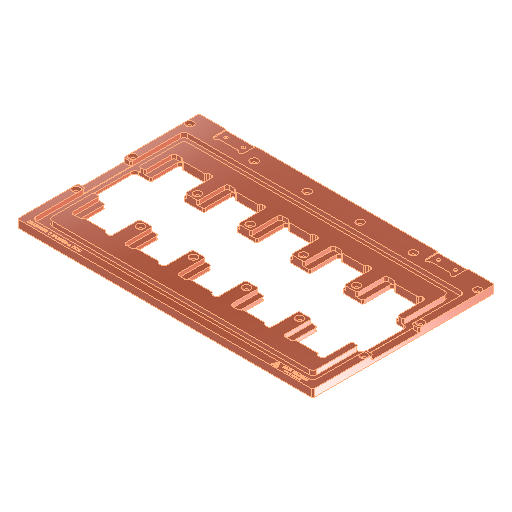
# Autodesk Inventor part: GRJ-04-104
Saved by Autodesk Inventor 2026.1 (Build 301233000, 233)
## iProperties
Company: Gree
Created: 2025-09-10
Part Number: GRJ-04-104
Material: Fenolite OR
Document SubType Name: Modeling
Designer: Willian Pinheiro
Density: 1.38 g/cm^3
Appearance: Suave - Laranja claro
Description: Suporte Dissipador G GRJW890-A
Project: GRJ-04
Mass: 640.909 g
Surface Area: 1542.93 cm^2
Volume: 464.426 cm^3
Checked By: Antonio Lucas
Engr Approved By: Antonio Lucas
Mfg Approved By: Anderson Oliveira
Total: 1
Dimensões: 10 x 240 x 390 mm
Author: Willian Pinheiro
Title: Pasta Dissipador G
Revision Number: 00
Autodesk Inventor part; units mm, degrees
(part 1 of 3)
sketch "comp_ipm-d5-g1-db2" plane through (0, 0, 0) normal (0, 0, 1) x (1, 0, 0)
  line L0 (114.3417, -62.3123) -> (114.3417, -51.4863) construction
  line L1 (114.3417, -51.4863) -> (133.7146, -51.4863) construction
  line L2 (133.611, -89.7496) -> (133.611, -119.2687) construction
  line L3 (133.611, -119.2687) -> (119.4922, -119.2687) construction
  line L4 (119.4922, -119.2687) -> (119.4922, -89.8381) construction
  line L5 (119.4922, -89.8381) -> (119.5805, -89.7496) construction
  line L6 (119.5805, -89.7496) -> (133.611, -89.7496) construction
  line L7 (122.7317, -8.8892) -> (130.2416, -8.8892) construction
  line L8 (133.3346, -81.6323) -> (111.2285, -81.6323) construction
  line L9 (111.2285, -81.6323) -> (111.2285, -65.8863) construction
  line L10 (111.2285, -65.8863) -> (133.3346, -65.8863) construction
  line L11 (133.3346, -65.8863) -> (133.3346, -81.6323) construction
  line L12 (130.2416, -8.8892) -> (130.2416, -41.4312) construction
  line L13 (130.2416, -41.4312) -> (122.7296, -41.4312) construction
  circle A0 centre (120.8945, -10.3261) radius 5 construction
  circle A1 centre (120.8747, -40.1261) radius 5 construction
  arc A2 (122.7096, -57.0141) -> (122.7172, -56.7385) centre (127.7095, -57.0141) ccw construction
  circle A3 centre (127.6714, -73.8746) radius 5 construction
  circle A4 centre (124.6717, -104.6746) radius 5 construction
  line L14 (122.7296, -41.4312) -> (122.7296, -40.059) construction
  arc A5 (122.7296, -40.0576) -> (119.2755, -40.047) centre (121.0027, -40.0154) ccw construction
  line L15 (119.2755, -40.047) -> (119.2755, -41.4312) construction
  line L16 (119.2755, -41.4312) -> (112.2015, -41.4312) construction
  line L17 (112.2015, -41.4312) -> (112.2015, -8.8892) construction
  line L18 (112.2015, -8.8892) -> (119.2755, -8.8892) construction
  line L19 (119.2755, -8.8892) -> (119.2755, -10.254) construction
  arc A6 (119.2755, -10.254) -> (119.2755, -10.1681) centre (121.0022, -10.211) ccw construction
  line L20 (122.7317, -10.1612) -> (122.7317, -8.8892) construction
  circle A7 centre (127.8416, -56.8993) radius 5.127 construction
  line L21 (133.7146, -51.4863) -> (133.7146, -62.3123) construction
  line L22 (133.7146, -62.3123) -> (114.3417, -62.3123) construction
sketch "dissi-g-grjw890-a(v1.6)" plane through (0, 0, 0) normal (0, 0, 1) x (1, 0, 0)
  line L0 (-21.5, -6.5) -> (-21.5, 123.5) construction
  line L1 (31, -6.5) -> (-21.5, -6.5) construction
  line L2 (-21.5, -1.5) -> (31, -1.5) construction
  line L3 (31, -4.5) -> (-21.5, -4.5) construction
  line L4 (31, -6.5) -> (31, 123.5) construction
  line L5 (-21.5, 121.5) -> (31, 121.5) construction
  line L6 (20.379, 118.5) -> (-21.5, 118.5) construction
  line L7 (31, 118.5) -> (23.621, 118.5) construction
  arc A0 (23.621, 118.5) -> (20.379, 118.5) centre (22, 118.5) ccw construction
  arc A1 (20.379, 118.5) -> (23.621, 118.5) centre (22, 118.5) ccw construction
  line L8 (-21.5, 123.5) -> (31, 123.5) construction
  circle A2 centre (9.1772, 15.1514) radius 1.2295 construction
  circle A3 centre (12.177, 45.9515) radius 1.2295 construction
  circle A4 centre (12.3472, 62.9268) radius 1.2295 construction
  circle A5 centre (5.5082, 79.8107) radius 1.2295 construction
  circle A6 centre (5.4, 109.5) radius 1.2295 construction
  arc A7 (0, 71.9528) -> (-1.2857, 75.3) centre (-5, 71.9528) ccw construction
  line L9 (0, 71.9528) -> (0, 0) construction
  line L10 (0, 0) -> (19.4, 0) construction
  line L11 (19.4, 0) -> (19.4, 69.7008) construction
  arc A8 (19.4, 69.7008) -> (17.4571, 71.7) centre (17.4, 69.7008) ccw construction
  arc A9 (12.6, 76.698) -> (17.4571, 71.7) centre (17.6, 76.698) ccw construction
  line L12 (12.6, 76.698) -> (12.6, 113.5) construction
  line L13 (12.6, 113.5) -> (-1.8, 113.5) construction
  line L14 (-1.8, 113.5) -> (-1.8, 76.6389) construction
  arc A10 (-1.8, 76.6389) -> (-1.2857, 75.3) centre (0.2, 76.6389) ccw construction
  circle A11 centre (5.4, 109.5) radius 1.2295 construction
  circle A12 centre (5.5082, 79.8107) radius 1.2295 construction
  line L15 (-14, 123.5) -> (-14, -6.5) construction
  line L16 (28.5, 123.5) -> (28.5, -6.5) construction
  line L17 (-21.5, 58.5) -> (31, 58.5) construction
  line L18 (-1.1528, 57.5138) -> (-1.1528, 68.3398) construction
  line L19 (-1.1528, 68.3398) -> (18.2202, 68.3398) construction
  line L20 (18.1165, 30.0765) -> (18.1165, 0.5573) construction
  line L21 (18.1165, 0.5573) -> (3.9977, 0.5573) construction
  line L22 (3.9977, 0.5573) -> (3.9977, 29.988) construction
  line L23 (3.9977, 29.988) -> (4.0861, 30.0765) construction
  line L24 (4.0861, 30.0765) -> (18.1165, 30.0765) construction
  line L25 (7.2372, 110.9369) -> (14.7471, 110.9369) construction
  line L26 (17.8402, 38.1938) -> (-4.266, 38.1938) construction
  line L27 (-4.266, 38.1938) -> (-4.266, 53.9398) construction
  line L28 (-4.266, 53.9398) -> (17.8402, 53.9398) construction
  line L29 (17.8402, 53.9398) -> (17.8402, 38.1938) construction
  line L30 (14.7471, 110.9369) -> (14.7471, 78.3949) construction
  line L31 (14.7471, 78.3949) -> (7.2352, 78.3949) construction
  circle A13 centre (5.4, 109.5) radius 5 construction
  circle A14 centre (5.3802, 79.6999) radius 5 construction
  arc A15 (7.2151, 62.812) -> (7.2227, 63.0876) centre (12.2151, 62.812) ccw construction
  circle A16 centre (12.177, 45.9515) radius 5 construction
  circle A17 centre (9.1772, 15.1514) radius 5 construction
  line L32 (7.2352, 78.3949) -> (7.2352, 79.7671) construction
  arc A18 (7.2352, 79.7685) -> (3.781, 79.779) centre (5.5082, 79.8107) ccw construction
  line L33 (3.781, 79.779) -> (3.781, 78.3949) construction
  line L34 (3.781, 78.3949) -> (-3.293, 78.3949) construction
  line L35 (-3.293, 78.3949) -> (-3.293, 110.9369) construction
  line L36 (-3.293, 110.9369) -> (3.781, 110.9369) construction
  line L37 (3.781, 110.9369) -> (3.781, 109.5721) construction
  arc A19 (3.781, 109.5721) -> (3.781, 109.658) centre (5.5077, 109.615) ccw construction
  line L38 (7.2372, 109.6648) -> (7.2372, 110.9369) construction
  circle A20 centre (12.3472, 62.9268) radius 5.127 construction
  line L39 (18.2202, 68.3398) -> (18.2202, 57.5138) construction
  line L40 (18.2202, 57.5138) -> (-1.1528, 57.5138) construction
  dimension "d211" = 7.5
  dimension "d212" = 2.5
  measures "d211" distance between parallel lines of L0 L15
  measures "d212" distance between parallel lines of L4 L16
sketch "Logo-Delta" plane through (0, 0, 0) normal (0, 0, 1) x (1, 0, 0)
  line L0 (-108.5421, -93.8239) -> (-105.2306, -99.7477)
  line L1 (-105.8771, -100.8237) -> (-112.693, -100.8237)
  line L2 (-113.3004, -99.7477) -> (-112.693, -100.8237)
  line L3 (-109.8866, -93.8239) -> (-113.3004, -99.7477)
  line L4 (-109.8866, -93.8239) -> (-108.5421, -93.8239)
  line L5 (-108.6943, -94.0618) -> (-109.6978, -94.0618)
  line L6 (-107.1297, -98.6558) -> (-109.869, -98.6558)
  line L7 (-110.3581, -99.4928) -> (-105.6768, -99.4597)
  line L8 (-108.6943, -94.0618) -> (-105.6768, -99.4597)
  line L9 (-107.5019, -98.4356) -> (-108.4992, -98.4356)
  line L10 (-109.8866, -96.0618) -> (-112.5468, -100.5747)
  line L11 (-112.9983, -99.775) -> (-109.8866, -94.3555)
  line L12 (-109.869, -98.6558) -> (-110.3581, -99.4928)
  line L13 (-109.8866, -94.3555) -> (-107.5019, -98.4356)
  line L14 (-109.6978, -94.0618) -> (-109.6206, -94.2)
  line L15 (-109.8866, -96.0618) -> (-108.4992, -98.4356)
  line L16 (-109.6978, -94.0618) -> (-107.1297, -98.6558)
  line L17 (-112.9983, -99.775) -> (-112.5468, -100.5747)
  line L18 (-105.2306, -99.7477) -> (-105.8771, -100.8237)
  line L19 (-109.3597, -97.315) -> (-110.8037, -99.7825)
  line L20 (-110.8037, -99.7825) -> (-105.5116, -99.7553)
  line L21 (-105.5116, -99.7553) -> (-105.978, -100.5522)
  line L22 (-105.978, -100.5522) -> (-112.2705, -100.5522)
  line L23 (-112.2705, -100.5522) -> (-109.8735, -96.4562)
  line L24 (-109.2558, -97.6251) -> (-109.7424, -98.4356)
  line L25 (-109.7424, -98.4356) -> (-108.7692, -98.4356)
  line L26 (-108.7692, -98.4356) -> (-109.2558, -97.6251)
  line L27 (-109.8735, -96.4562) -> (-109.3597, -97.315)
  line L28 (-109.2558, -97.6251) -> (-108.7692, -98.4356)
  point P0 (-109.285, -100.8237)
  dimension "d228" = 33
  dimension "d229" = 50
  dimension "d230" = 5
  dimension "d231" = 9
  dimension "d232" = 2.5
  dimension "d233" = 6
  dimension "d234" = 150
  dimension "d235" = 12
  dimension "d236" = 15
  dimension "d237" = 13.4
  dimension "d238" = 5.5006
  dimension "d239" = 12.9994
  dimension "d240" = 12.9994
  dimension "d227" = 7
sketch "Esboço1" plane through (0, 0, 0) normal (0, 0, 1) x (1, 0, 0)
  line L0 (-195, 130) -> (195, 130)
  line L1 (195, 130) -> (195, -110)
  line L2 (195, -110) -> (-195, -110)
  line L3 (-195, -110) -> (-195, 130)
  line L4 (0, 179.4497) -> (0, -159.4497) construction
  line L5 (-274.4497, 0) -> (274.4497, 0) construction
  arc A0 (-190, 130) -> (-195, 125) centre (-190, 125) ccw
  arc A1 (195, 125) -> (190, 130) centre (190, 125) ccw
  arc A2 (190, -110) -> (195, -105) centre (190, -105) ccw
  arc A3 (-195, -105) -> (-190, -110) centre (-190, -105) ccw
  line L6 (-165, 0) -> (-65, 0) construction
  line L7 (-113.55, 65.2) -> (-166.45, 65.2)
  line L8 (-166.45, 65.2) -> (-166.45, -65.2)
  line L9 (-166.45, -65.2) -> (-113.55, -65.2)
  line L10 (-113.55, -65.2) -> (-113.55, 65.2)
  line L11 (-116.05, 65.2) -> (-158.95, 65.2)
  line L12 (-158.95, 65.2) -> (-158.95, -65.2)
  line L13 (-158.95, -65.2) -> (-116.05, -65.2)
  line L14 (-116.05, -65.2) -> (-116.05, 65.2)
  line L15 (-158.95, 0) -> (-116.05, 0) construction
  line L16 (-195, 30) -> (195, 30)
  line L17 (195, 30) -> (195, -30)
  line L18 (195, -30) -> (-195, -30)
  line L19 (-195, -30) -> (-195, 30)
  line L20 (-175, 90) -> (175, 90) construction
  line L21 (175, 90) -> (175, -90) construction
  line L22 (175, -90) -> (-175, -90) construction
  line L23 (-175, -90) -> (-175, 90) construction
  line L24 (-185, 100) -> (185, 100) construction
  line L25 (185, 100) -> (185, -100) construction
  line L26 (185, -100) -> (-185, -100) construction
  line L27 (-185, -100) -> (-185, 100) construction
  line L28 (185.4, 100.4) -> (-185.4, 100.4)
  line L29 (-185.4, 100.4) -> (-185.4, -100.4)
  line L30 (-185.4, -100.4) -> (185.4, -100.4)
  line L31 (185.4, -100.4) -> (185.4, 100.4)
  line L32 (174.6, 89.6) -> (-174.6, 89.6)
  line L33 (-174.6, 89.6) -> (-174.6, -89.6)
  line L34 (-174.6, -89.6) -> (174.6, -89.6)
  line L35 (174.6, -89.6) -> (174.6, 89.6)
  line L36 (-159.5, 130) -> (-120.5, 130)
  line L37 (-120.5, 130) -> (-120.5, 114)
  line L38 (-120.5, 114) -> (-159.5, 114)
  line L39 (-159.5, 114) -> (-159.5, 130)
  circle A4 centre (-156.5, 114) radius 3
  line L40 (-140, 114) -> (-140, 130) construction
  line L41 (-159.5, 122) -> (-120.5, 122) construction
  circle A5 centre (-123.5, 114) radius 3
  line L42 (159.5, 130) -> (120.5, 130)
  line L43 (120.5, 130) -> (120.5, 114)
  line L44 (120.5, 114) -> (159.5, 114)
  line L45 (159.5, 114) -> (159.5, 130)
  circle A6 centre (156.5, 114) radius 3
  line L46 (140, 114) -> (140, 130) construction
  line L47 (159.5, 122) -> (120.5, 122) construction
  circle A7 centre (123.5, 114) radius 3
  line L48 (-195, 10) -> (195, 10) construction
  line L49 (-180, 30) -> (-180, -30)
  line L50 (180, 30) -> (180, -30)
  line L51 (-140, 65) -> (-140, -65) construction
  line L52 (-105, 89.6) -> (-105, -100.4) construction
  line L53 (-70, 65) -> (-70, -65) construction
  line L54 (140, 65) -> (140, -65) construction
  line L55 (70, 65) -> (70, -65) construction
  circle A8 centre (-163.45, 65.2) radius 3
  circle A9 centre (-119.05, 65.2) radius 3
  circle A10 centre (-155.95, 65.2) radius 3
  circle A11 centre (-116.55, 65.2) radius 3
  circle A12 centre (-163.45, -65.2) radius 3
  circle A13 centre (-119.05, -65.2) radius 3
  circle A14 centre (-155.95, -65.2) radius 3
  circle A15 centre (-116.55, -65.2) radius 3
  line L56 (-163.45, 68.2) -> (-155.95, 68.2)
  line L57 (-116.55, 68.2) -> (-119.05, 68.2)
  line L58 (-163.45, -68.2) -> (-155.95, -68.2)
  line L59 (-119.05, -68.2) -> (-116.55, -68.2)
  line L60 (-166.25, -65) -> (-166.25, 65) construction
  line L61 (-113.75, -65) -> (-166.25, -65) construction
  line L62 (-166.25, -60) -> (-113.75, -60) construction
  line L63 (-113.75, -63) -> (-166.25, -63) construction
  line L64 (-113.75, -65) -> (-113.75, 65) construction
  line L65 (-166.25, 63) -> (-113.75, 63) construction
  line L66 (-124.371, 60) -> (-166.25, 60) construction
  line L67 (-113.75, 60) -> (-121.129, 60) construction
  arc A16 (-121.129, 60) -> (-124.371, 60) centre (-122.75, 60) ccw construction
  arc A17 (-124.371, 60) -> (-121.129, 60) centre (-122.75, 60) ccw construction
  line L68 (-166.25, 65) -> (-113.75, 65) construction
  circle A18 centre (-135.5728, -43.3486) radius 1.2295 construction
  circle A19 centre (-132.573, -12.5485) radius 1.2295 construction
  circle A20 centre (-132.4028, 4.4268) radius 1.2295 construction
  circle A21 centre (-139.2418, 21.3107) radius 1.2295 construction
  circle A22 centre (-139.35, 51) radius 1.2295 construction
  arc A23 (-144.75, 13.4528) -> (-146.0357, 16.8) centre (-149.75, 13.4528) ccw construction
  line L69 (-144.75, 13.4528) -> (-144.75, -58.5) construction
  line L70 (-144.75, -58.5) -> (-125.35, -58.5) construction
  line L71 (-125.35, -58.5) -> (-125.35, 11.2008) construction
  arc A24 (-125.35, 11.2008) -> (-127.2929, 13.2) centre (-127.35, 11.2008) ccw construction
  arc A25 (-132.15, 18.198) -> (-127.2929, 13.2) centre (-127.15, 18.198) ccw construction
  line L72 (-132.15, 18.198) -> (-132.15, 55) construction
  line L73 (-132.15, 55) -> (-146.55, 55) construction
  line L74 (-146.55, 55) -> (-146.55, 18.1389) construction
  arc A26 (-146.55, 18.1389) -> (-146.0357, 16.8) centre (-144.55, 18.1389) ccw construction
  circle A27 centre (-139.35, 51) radius 1.2295 construction
  circle A28 centre (-139.2418, 21.3107) radius 1.2295 construction
  line L75 (-158.75, 65) -> (-158.75, -65) construction
  line L76 (-116.25, 65) -> (-116.25, -65) construction
  line L77 (-166.25, 0) -> (-113.75, 0) construction
  line L78 (-145.9028, -0.9862) -> (-145.9028, 9.8398) construction
  line L79 (-145.9028, 9.8398) -> (-126.5298, 9.8398) construction
  line L80 (-126.6335, -28.4235) -> (-126.6335, -57.9427) construction
  line L81 (-126.6335, -57.9427) -> (-140.7523, -57.9427) construction
  line L82 (-140.7523, -57.9427) -> (-140.7523, -28.512) construction
  line L83 (-140.7523, -28.512) -> (-140.6639, -28.4235) construction
  line L84 (-140.6639, -28.4235) -> (-126.6335, -28.4235) construction
  line L85 (-137.5128, 52.4369) -> (-130.0029, 52.4369) construction
  line L86 (-126.9098, -20.3062) -> (-149.016, -20.3062) construction
  line L87 (-149.016, -20.3062) -> (-149.016, -4.5602) construction
  line L88 (-149.016, -4.5602) -> (-126.9098, -4.5602) construction
  line L89 (-126.9098, -4.5602) -> (-126.9098, -20.3062) construction
  line L90 (-130.0029, 52.4369) -> (-130.0029, 19.8949) construction
  line L91 (-130.0029, 19.8949) -> (-137.5148, 19.8949) construction
  circle A29 centre (-139.35, 51) radius 5 construction
  circle A30 centre (-139.3698, 21.1999) radius 5 construction
  arc A31 (-137.5349, 4.312) -> (-137.5273, 4.5876) centre (-132.5349, 4.312) ccw construction
  circle A32 centre (-132.573, -12.5485) radius 5 construction
  circle A33 centre (-135.5728, -43.3486) radius 5 construction
  line L92 (-137.5148, 19.8949) -> (-137.5148, 21.2671) construction
  arc A34 (-137.5148, 21.2685) -> (-140.969, 21.279) centre (-139.2418, 21.3107) ccw construction
  line L93 (-140.969, 21.279) -> (-140.969, 19.8949) construction
  line L94 (-140.969, 19.8949) -> (-148.043, 19.8949) construction
  line L95 (-148.043, 19.8949) -> (-148.043, 52.4369) construction
  line L96 (-148.043, 52.4369) -> (-140.969, 52.4369) construction
  line L97 (-140.969, 52.4369) -> (-140.969, 51.0721) construction
  arc A35 (-140.969, 51.0721) -> (-140.969, 51.158) centre (-139.2423, 51.115) ccw construction
  line L98 (-137.5128, 51.1648) -> (-137.5128, 52.4369) construction
  circle A36 centre (-132.4028, 4.4268) radius 5.127 construction
  line L99 (-126.5298, 9.8398) -> (-126.5298, -0.9862) construction
  line L100 (-126.5298, -0.9862) -> (-145.9028, -0.9862) construction
  point P0 (0, 0)
  point P1 (-151.5, 122)
  point P2 (-128.5, 122)
  point P3 (151.5, 122)
  point P4 (128.5, 122)
  point P5 (-190, 37.5)
  point P6 (-190, -37.5)
  point P7 (190, 37.5)
  point P8 (190, -37.5)
  point P9 (-190, 112.5)
  point P10 (190, 112.5)
  point P11 (-35, 37.5)
  point P12 (-35, -37.5)
  point P13 (-35, 112.5)
  point P14 (35, 37.5)
  point P15 (35, -37.5)
  point P16 (35, 112.5)
  point P17 (120.5, 114)
  point P18 (126.5, 114)
  point P19 (153.5, 114)
  point P20 (159.5, 130)
  point P21 (120.5, 130)
  point P22 (-120.5, 114)
  point P23 (-120.5, 130)
  point P24 (-153.5, 114)
  point P25 (-126.5, 114)
  point P26 (-185.4, -30)
  point P27 (185.4, -30)
  point P28 (185.4, 30)
  point P29 (-185.4, 30)
  point P30 (-174.6, 30)
  point P31 (-174.6, -30)
  point P32 (174.6, -30)
  point P33 (174.6, 30)
  point P34 (-160.45, -65.2)
  point P35 (-119.55, -65.2)
  point P36 (-119.55, 65.2)
  point P37 (-160.45, 65.2)
  point P38 (-152.95, 65.2)
  point P39 (-152.95, -65.2)
  point P40 (-122.05, -65.2)
  point P41 (-122.05, 65.2)
  point P42 (-105, 37.5)
  point P43 (-105, -37.5)
  point P44 (-105, 112.5)
  point P45 (105, 37.5)
  point P46 (105, 112.5)
  point P47 (105, -37.5)
  dimension "d210" = 6
  dimension "d0" = 390
  dimension "d1" = 240
  dimension "d2" = 5
  dimension "d145" = 110
  dimension "d151" = 60
  dimension "d153" = 20
  dimension "d154" = 20
  dimension "d155" = 40
  dimension "d156" = 10
  dimension "d157" = 0.4
  dimension "d158" = 0.4
  dimension "d159" = 39
  dimension "d160" = 16
  dimension "d161" = 8
  dimension "d162" = 23
  dimension "d163" = 280
  dimension "d164" = 75
  dimension "d165" = 5
  dimension "d166" = 75
  dimension "d167" = 70
  dimension "d218" = 70
  dimension "d219" = 70
  dimension "d220" = 0.2
  dimension "d221" = 0.2
  dimension "d222" = 0.2
  dimension "d223" = 0.2
  constraints: 116 end point, 36 symmetric about line, 24 point on line, 18 parallel, 11 perpendicular, 10 horizontal, 10 midpoint, 8 point on circle, 8 tangent, 7 vertical alignment, 6 centre point, 5 vertical, 3 collinear, 3 equal radius, 3 horizontal alignment, 50 other
  measures "d0" distance of L0.start L0.end
  measures "d1" distance of L0.start L2.end
  measures "d2" radius of A0
  measures "d145" distance between parallel lines of L2 L5
  measures "d151" distance between parallel lines of L18 L16
  measures "d153" distance between parallel lines of L23 L3
  measures "d154" distance between parallel lines of L2 L22
  measures "d155" distance between parallel lines of L20 L0
  measures "d156" distance between parallel lines of L23 L27
  measures "d157" distance between parallel lines of L31 L25
  measures "d158" distance between parallel lines of L21 L35
  measures "d159" distance between parallel lines of L37 L39
  measures "d160" distance between parallel lines of L0 L38
  measures "d161" distance between parallel lines of L41 L36
  measures "d162" distance of point (-128.5, 122) point (-151.5, 122)
  measures "d163" distance between parallel lines of L40 L46
  measures "d164" distance of point (-190, 37.5) point (-190, -37.5)
  measures "d165" distance from line of L3 point (-190, -37.5)
  measures "d166" distance of point (-190, 112.5) point (-190, 37.5)
  measures "d167" distance of point (35, 112.5) point (-35, 112.5)
  measures "d218" distance between parallel lines of L4 L53
  measures "d219" distance between parallel lines of L51 L53
extrude "Extrusão1" add sketch "Esboço1" against normal blind 10
extrude "Extrusion22" cut sketch "Esboço1" against normal blind 1.3 contours L0 L37 A5 L38 A4 L39 | A4 L38 | L38 A4 | L0 L45 A6 L44 A7 L43 | A5 L38 | L38 A5 | A7 L44 | L44 A7 | A6 L44 | L44 A6
extrude "Extrusion23" cut sketch "Esboço1" against normal blind 6.1 contours L29 L28 L31 L16 L35 L32 L33 | L16 L49 L18 L29 | L18 L33 L34 L35 L31 L30 L29 | L16 L33 L18 L49 | L31 L18 L50 L16 | L50 L18 L35 L16
extrude "Extrusion24" cut sketch "Esboço1" against normal blind 5.4 contours L16 L29 L18 L3 | L16 L12 L18 L8 | L8 A8 L7 L12 L16 | L16 L1 L18 L31 | L18 L12 L9 A12 L8 | A8 L7 | L7 A8 | L16 L14 L18 L12 | L12 A10 L7 A9 A11 L14 L16 | A12 L9 | L9 A12 | L18 L14 A15 A13 L9 A14 L12 | A8 L56 A10 L7 | A10 L7 | L7 A10 | L16 L10 L18 L14 | L14 A11 L10 L16 | L9 A14 L58 A12 | A14 L9 | L9 A14 | L18 L10 A15 L14 | A11 A9 L14 | L14 L7 A11 | A15 L9 L14 | L14 A13 A15 | A9 A11 L7 | L7 A11 A9 | A9 A11 L7 | A9 A11 L7 | L7 A11 A9 | A13 A15 L9 | L9 A15 A13 | A13 A15 L9 | L9 A15 A13 | L9 A15 A13 | L57 A11 A9 | A13 A15 L59
extrude "Extrusion25" cut sketch "Esboço1" against normal through all contours L16 L14 L18 L12 | L12 A10 L7 A9 A11 L14 L16 | L18 L14 A15 A13 L9 A14 L12 | A10 L7 | L7 A10 | A14 L9 | L9 A14 | A11 A9 L14 | L14 A13 A15 | A9 A11 L7 | L7 A11 A9 | A9 A11 L7 | L7 A11 A9 | A13 A15 L9 | L9 A15 A13 | A13 A15 L9 | L9 A15 A13 picked at (-120.3323, 65.6487) picked at (-120.3328, 64.7533) picked at (-117.2426, 64.9738) picked at (-117.2426, 65.4262) picked at (-120.3328, -64.7533) picked at (-120.3323, -65.6487) picked at (-118.3574, -65.4262) picked at (-117.2426, -64.9738)
pattern_linear "Rectangular Pattern4" count 5 spacing 70 along (1, 0, 0) of "Extrusion24", "Extrusion25"
extrude "Extrusion26" cut sketch "Esboço1" against normal through all contours L16 L33 L18 L49 | L16 L8 L18 L33 | L16 L12 L18 L8 | L16 L14 L18 L12 | L50 L18 L35 L16 | L16 L10 L18 L14 | L35 L18 L10 L16
hole "Hole3" at (-151.5, 122, 0) at (-128.5, 122, 0) at (128.5, 122, 0) at (151.5, 122, 0) direction (0, 0, -1) diameter 2.459 end through all thread size "M3x0.5" class "6H" standard "ISO Metric profile"
hole "Hole4" at (-190, 37.5, 0) at (-190, -37.5, 0) at (190, 37.5, 0) at (190, -37.5, 0) at (-190, 112.5, 0) at (190, 112.5, 0) at (-35, 37.5, 0) at (-35, -37.5, 0) at (-35, 112.5, 0) at (35, 37.5, 0) at (35, 112.5, 0) at (35, -37.5, 0) at (-105, 112.5, 0) at (-105, 37.5, 0) at (-105, -37.5, 0) at (105, -37.5, 0) at (105, 37.5, 0) at (105, 112.5, 0) direction (0, 0, -1) diameter 4.5 end through all countersink diameter 10 countersink angle 90 clearance for "Countersunk Flat Head Hex Socket Screw ISO 10642" size "M4" standard "ISO"
fillet "Fillet10" radius 2 84 edges at (-113.55, 30, -2.7) (-96.45, 30, -2.7) (-113.55, -30, -2.7) (-96.45, -30, -2.7) (-43.55, 30, -2.7) (-26.45, 30, -2.7) (-26.45, -30, -2.7) (-43.55, -30, -2.7) (26.45, -30, -2.7) (174.6, -30, -3.05) (174.6, 30, -3.05) (26.45, 30, -2.7) (-166.45, -30, -2.7) (-174.6, -30, -3.05) (-153.5, 114, -0.65) (-126.5, 114, -0.65) (126.5, 114, -0.65) (153.5, 114, -0.65) (-174.6, 30, -3.05) (-166.45, 30, -2.7) (-195, 30, -2.7) (-185.4, 30, -2.7) (-195, -30, -2.7) (-185.4, -30, -2.7) (185.4, 30, -2.7) (195, 30, -2.7) (185.4, -30, -2.7) (195, -30, -2.7) (195, 130, -5) (195, -110, -5) (-195, -110, -5) (-195, 130, -5) (-152.95, 65.2, -5) (-122.05, 65.2, -5) (-116.05, 30, -7.7) (-158.95, 30, -7.7) (-88.95, 30, -7.7) (-82.95, 65.2, -5) (-52.05, 65.2, -5) (-46.05, 30, -7.7) (-18.95, 30, -7.7) (-12.95, 65.2, -5) (17.95, 65.2, -5) (23.95, 30, -7.7) (51.05, 30, -7.7) (57.05, 65.2, -5) (87.95, 65.2, -5) (93.95, 30, -7.7) (96.45, 30, -2.7) (43.55, 30, -2.7) (113.55, 30, -2.7) (121.05, 30, -7.7) (127.05, 65.2, -5) (157.95, 65.2, -5) (163.95, 30, -7.7) (166.45, 30, -2.7) (166.45, -30, -2.7) (163.95, -30, -7.7) (113.55, -30, -2.7) (121.05, -30, -7.7) (93.95, -30, -7.7) (96.45, -30, -2.7) (127.05, -65.2, -5) (157.95, -65.2, -5) (87.95, -65.2, -5) (57.05, -65.2, -5) (51.05, -30, -7.7) (43.55, -30, -2.7) (23.95, -30, -7.7) (17.95, -65.2, -5) (-12.95, -65.2, -5) (-18.95, -30, -7.7) (-46.05, -30, -7.7) (-88.95, -30, -7.7) (-116.05, -30, -7.7) (-158.95, -30, -7.7) (-152.95, -65.2, -5) (-122.05, -65.2, -5) (-82.95, -65.2, -5) (-52.05, -65.2, -5) (-159.5, 130, -0.65) (-120.5, 130, -0.65) (120.5, 130, -0.65) (159.5, 130, -0.65)
fillet "Fillet10" radius 5 12 edges at (174.6, -89.6, -3.05) (185.4, -100.4, -3.05) (-185.4, -100.4, -3.05) (-174.6, -89.6, -3.05) (-185.4, 100.4, -3.05) (-174.6, 89.6, -3.05) (185.4, 100.4, -3.05) (174.6, 89.6, -3.05) (-180, 30, -8.05) (-180, -30, -8.05) (180, -30, -8.05) (180, 30, -8.05)
chamfer "Chamfer3" [suppressed]
chamfer "Chamfer4" distance 1 angle 45 4 edges at (-151.5, 123.2295, -1.3) (-128.5, 123.2295, -1.3) (128.5, 123.2295, -1.3) (151.5, 123.2295, -1.3)
ref_plane "Work Plane1" through (-140, 65.2, 0) normal (1, 0, 0) x (0, 0, -1)
ref_plane "Work Plane2" through (-70, 65.2, 0) normal (1, 0, 0) x (0, 0, -1)
ref_plane "Work Plane3" through (0, 65.2, 0) normal (1, 0, 0) x (0, 0, -1)
ref_plane "Plano de trabalho4" through (70, 65.2, 0) normal (1, 0, 0) x (0, 0, -1)
ref_plane "Plano de trabalho5" through (140, 65.2, 0) normal (1, 0, 0) x (0, 0, -1)
sketch "Esboço27" plane through (0, 0, 0) normal (0, 0, 1) x (1, 0, 0)
  line L0 (-185.4, -107) -> (-185.4, -103) construction
  line L1 (-185.4, -103) -> (-2.1339, -103) construction
  line L2 (-2.1339, -103) -> (-2.1339, -107) construction
  line L3 (-2.1339, -107) -> (-185.4, -107) construction
  line L4 (-193, -110) -> (193, -110) projected
  line L5 (-195, -37.5) -> (-195, -108) projected
  line L6 (145.4, -108.5) -> (145.4, -101.5) construction
  line L7 (148.9, -108.5) -> (148.9, -104.5) construction
  line L8 (165.4, -101.5) -> (165.4, -108.5) construction
  line L9 (181.9, -104.5) -> (181.9, -108.5) construction
  line L10 (148.9, -104.5) -> (181.9, -104.5) construction
  line L11 (181.9, -108.5) -> (148.9, -108.5) construction
  line L12 (185.4, -108.5) -> (145.4, -108.5) construction
  line L13 (185.4, -101.5) -> (185.4, -108.5) construction
  line L14 (145.4, -101.5) -> (185.4, -101.5) construction
  line L15 (185.4, -39.4596) -> (185.4, -95.4) construction
  line L16 (-185.4, -95.4) -> (-185.4, -39.4596) projected
  line L17 (143.0723, -101.5) -> (146.3837, -107.4238)
  line L18 (145.7373, -108.4998) -> (138.9214, -108.4998)
  line L19 (138.3139, -107.4238) -> (138.9214, -108.4998)
  line L20 (141.7277, -101.5) -> (138.3139, -107.4238)
  line L21 (141.7277, -101.5) -> (143.0723, -101.5)
  line L22 (142.9201, -101.7378) -> (141.9165, -101.7378)
  line L23 (144.4846, -106.3319) -> (141.7453, -106.3319)
  line L24 (141.2562, -107.1689) -> (145.9375, -107.1357)
  line L25 (142.9201, -101.7378) -> (145.9375, -107.1357)
  line L26 (144.1124, -106.1117) -> (143.1151, -106.1117)
  line L27 (141.7277, -103.7379) -> (139.0676, -108.2507)
  line L28 (138.6161, -107.451) -> (141.7277, -102.0316)
  line L29 (141.7453, -106.3319) -> (141.2562, -107.1689)
  line L30 (141.7277, -102.0316) -> (144.1124, -106.1117)
  line L31 (141.9165, -101.7378) -> (141.9938, -101.8761)
  line L32 (141.7277, -103.7379) -> (143.1151, -106.1117)
  line L33 (141.9165, -101.7378) -> (144.4846, -106.3319)
  line L34 (138.6161, -107.451) -> (139.0676, -108.2507)
  line L35 (146.3837, -107.4238) -> (145.7373, -108.4998)
  line L36 (142.2546, -104.991) -> (140.8106, -107.4586)
  line L37 (140.8106, -107.4586) -> (146.1027, -107.4314)
  line L38 (146.1027, -107.4314) -> (145.6364, -108.2283)
  line L39 (145.6364, -108.2283) -> (139.3439, -108.2283)
  line L40 (139.3439, -108.2283) -> (141.7409, -104.1323)
  line L41 (142.3585, -105.3012) -> (141.8719, -106.1117)
  line L42 (141.8719, -106.1117) -> (142.8452, -106.1117)
  line L43 (142.8452, -106.1117) -> (142.3585, -105.3012)
  line L44 (141.7409, -104.1323) -> (142.2546, -104.991)
  line L45 (142.3585, -105.3012) -> (142.8452, -106.1117)
  spline S0 degree 2 poles (-185.0494, -103.5227) (-185.0494, -103.3474) (-184.874, -103.3474) knots 0 0 0 1 1 1
  line L46 (-184.874, -103.3474) -> (-183.8253, -103.3474)
  spline S1 degree 2 poles (-183.8253, -103.3474) (-183.4584, -103.3474) (-182.9519, -103.8539) (-182.9519, -104.2208) knots 0 0 0 1 2 2 2
  line L47 (-182.9519, -104.2208) -> (-182.9519, -105.9708)
  spline S2 degree 2 poles (-182.9519, -105.9708) (-182.9519, -106.3344) (-183.4617, -106.8474) (-183.8253, -106.8474) knots 0 0 0 1 2 2 2
  line L48 (-183.8253, -106.8474) -> (-184.874, -106.8474)
  spline S3 degree 2 poles (-184.874, -106.8474) (-185.0494, -106.8474) (-185.0494, -106.6721) knots 0 0 0 1 1 1
  line L49 (-185.0494, -106.6721) -> (-185.0494, -103.5227)
  line L50 (-184.6987, -103.6981) -> (-184.6987, -106.4968)
  line L51 (-184.6987, -106.4968) -> (-183.8253, -106.4968)
  spline S4 degree 2 poles (-183.8253, -106.4968) (-183.6078, -106.4968) (-183.3026, -106.1883) (-183.3026, -105.9708) knots 0 0 0 1 2 2 2
  line L52 (-183.3026, -105.9708) -> (-183.3026, -104.224)
  spline S5 degree 2 poles (-183.3026, -104.224) (-183.3026, -104.0065) (-183.6078, -103.6981) (-183.8253, -103.6981) knots 0 0 0 1 2 2 2
  line L53 (-183.8253, -103.6981) -> (-184.6987, -103.6981)
  spline S6 degree 2 poles (-182.0753, -106.8474) (-182.2506, -106.8474) (-182.2506, -106.6721) knots 0 0 0 1 1 1
  line L54 (-182.2506, -106.6721) -> (-182.2506, -103.5227)
  spline S7 degree 2 poles (-182.2506, -103.5227) (-182.2506, -103.3474) (-182.0753, -103.3474) knots 0 0 0 1 1 1
  spline S8 degree 2 poles (-182.0753, -103.3474) (-181.9, -103.3474) (-181.9, -103.5227) knots 0 0 0 1 1 1
  line L55 (-181.9, -103.5227) -> (-181.9, -106.6721)
  spline S9 degree 2 poles (-181.9, -106.6721) (-181.9, -106.8474) (-182.0753, -106.8474) knots 0 0 0 1 1 1
  spline S10 degree 2 poles (-179.1045, -105.974) (-179.1045, -106.3344) (-179.6175, -106.8474) (-179.9779, -106.8474) knots 0 0 0 1 2 2 2
  spline S11 degree 2 poles (-179.9779, -106.8474) (-180.624, -106.8474) (-181.124, -106.4643) knots 0 0 0 1 1 1
  spline S12 degree 2 poles (-181.124, -106.4643) (-181.2019, -106.4058) (-181.2019, -106.3214) knots 0 0 0 1 1 1
  spline S13 degree 2 poles (-181.2019, -106.3214) (-181.2019, -106.25) (-181.0981, -106.1461) (-181.0266, -106.1461) knots 0 0 0 1 2 2 2
  spline S14 degree 2 poles (-181.0266, -106.1461) (-180.9844, -106.1461) (-180.926, -106.1786) knots 0 0 0 1 1 1
  spline S15 degree 2 poles (-180.926, -106.1786) (-180.7734, -106.2727) (-180.4455, -106.4221) knots 0 0 0 1 1 1
  spline S16 degree 2 poles (-180.4455, -106.4221) (-180.2312, -106.4968) (-179.9779, -106.4968) knots 0 0 0 1 1 1
  spline S17 degree 2 poles (-179.9779, -106.4968) (-179.7636, -106.4968) (-179.4552, -106.1883) (-179.4552, -105.9708) knots 0 0 0 1 2 2 2
  spline S18 degree 2 poles (-179.4552, -105.9708) (-179.4552, -105.6526) (-179.7474, -105.5032) knots 0 0 0 1 1 1
  line L56 (-179.7474, -105.5032) -> (-180.7279, -105)
  spline S19 degree 2 poles (-180.7279, -105) (-181.2019, -104.7565) (-181.2019, -104.2208) knots 0 0 0 1 1 1
  spline S20 degree 2 poles (-181.2019, -104.2208) (-181.2019, -103.8604) (-180.689, -103.3474) (-180.3286, -103.3474) knots 0 0 0 1 2 2 2
  spline S21 degree 2 poles (-180.3286, -103.3474) (-179.7084, -103.3474) (-179.3838, -103.539) knots 0 0 0 1 1 1
  spline S22 degree 2 poles (-179.3838, -103.539) (-179.2799, -103.6006) (-179.2799, -103.6981) knots 0 0 0 1 1 1
  spline S23 degree 2 poles (-179.2799, -103.6981) (-179.2799, -103.7695) (-179.3838, -103.8734) (-179.4552, -103.8734) knots 0 0 0 1 2 2 2
  spline S24 degree 2 poles (-179.4552, -103.8734) (-179.4812, -103.8734) (-179.5299, -103.8539) knots 0 0 0 1 1 1
  spline S25 degree 2 poles (-179.5299, -103.8539) (-179.9325, -103.6981) (-180.3286, -103.6981) knots 0 0 0 1 1 1
  spline S26 degree 2 poles (-180.3286, -103.6981) (-180.5461, -103.6981) (-180.8513, -104.0065) (-180.8513, -104.224) knots 0 0 0 1 2 2 2
  spline S27 degree 2 poles (-180.8513, -104.224) (-180.8513, -104.5422) (-180.5656, -104.6883) knots 0 0 0 1 1 1
  line L57 (-180.5656, -104.6883) -> (-179.5851, -105.1916)
  spline S28 degree 2 poles (-179.5851, -105.1916) (-179.1045, -105.4383) (-179.1045, -105.974) knots 0 0 0 1 1 1
  spline S29 degree 2 poles (-176.3058, -105.974) (-176.3058, -106.3344) (-176.8188, -106.8474) (-177.1792, -106.8474) knots 0 0 0 1 2 2 2
  spline S30 degree 2 poles (-177.1792, -106.8474) (-177.8253, -106.8474) (-178.3253, -106.4643) knots 0 0 0 1 1 1
  spline S31 degree 2 poles (-178.3253, -106.4643) (-178.4032, -106.4058) (-178.4032, -106.3214) knots 0 0 0 1 1 1
  spline S32 degree 2 poles (-178.4032, -106.3214) (-178.4032, -106.25) (-178.2994, -106.1461) (-178.2279, -106.1461) knots 0 0 0 1 2 2 2
  spline S33 degree 2 poles (-178.2279, -106.1461) (-178.1857, -106.1461) (-178.1273, -106.1786) knots 0 0 0 1 1 1
  spline S34 degree 2 poles (-178.1273, -106.1786) (-177.9747, -106.2727) (-177.6468, -106.4221) knots 0 0 0 1 1 1
  spline S35 degree 2 poles (-177.6468, -106.4221) (-177.4325, -106.4968) (-177.1792, -106.4968) knots 0 0 0 1 1 1
  spline S36 degree 2 poles (-177.1792, -106.4968) (-176.9649, -106.4968) (-176.6565, -106.1883) (-176.6565, -105.9708) knots 0 0 0 1 2 2 2
  spline S37 degree 2 poles (-176.6565, -105.9708) (-176.6565, -105.6526) (-176.9487, -105.5032) knots 0 0 0 1 1 1
  line L58 (-176.9487, -105.5032) -> (-177.9292, -105)
  spline S38 degree 2 poles (-177.9292, -105) (-178.4032, -104.7565) (-178.4032, -104.2208) knots 0 0 0 1 1 1
  spline S39 degree 2 poles (-178.4032, -104.2208) (-178.4032, -103.8604) (-177.8903, -103.3474) (-177.5299, -103.3474) knots 0 0 0 1 2 2 2
  spline S40 degree 2 poles (-177.5299, -103.3474) (-176.9097, -103.3474) (-176.5851, -103.539) knots 0 0 0 1 1 1
  spline S41 degree 2 poles (-176.5851, -103.539) (-176.4812, -103.6006) (-176.4812, -103.6981) knots 0 0 0 1 1 1
  spline S42 degree 2 poles (-176.4812, -103.6981) (-176.4812, -103.7695) (-176.5851, -103.8734) (-176.6565, -103.8734) knots 0 0 0 1 2 2 2
  spline S43 degree 2 poles (-176.6565, -103.8734) (-176.6825, -103.8734) (-176.7312, -103.8539) knots 0 0 0 1 1 1
  spline S44 degree 2 poles (-176.7312, -103.8539) (-177.1338, -103.6981) (-177.5299, -103.6981) knots 0 0 0 1 1 1
  spline S45 degree 2 poles (-177.5299, -103.6981) (-177.7474, -103.6981) (-178.0526, -104.0065) (-178.0526, -104.224) knots 0 0 0 1 2 2 2
  spline S46 degree 2 poles (-178.0526, -104.224) (-178.0526, -104.5422) (-177.7669, -104.6883) knots 0 0 0 1 1 1
  line L59 (-177.7669, -104.6883) -> (-176.7864, -105.1916)
  spline S47 degree 2 poles (-176.7864, -105.1916) (-176.3058, -105.4383) (-176.3058, -105.974) knots 0 0 0 1 1 1
  spline S48 degree 2 poles (-175.4292, -106.8474) (-175.6045, -106.8474) (-175.6045, -106.6721) knots 0 0 0 1 1 1
  line L60 (-175.6045, -106.6721) -> (-175.6045, -103.5227)
  spline S49 degree 2 poles (-175.6045, -103.5227) (-175.6045, -103.3474) (-175.4292, -103.3474) knots 0 0 0 1 1 1
  spline S50 degree 2 poles (-175.4292, -103.3474) (-175.2539, -103.3474) (-175.2539, -103.5227) knots 0 0 0 1 1 1
  line L61 (-175.2539, -103.5227) -> (-175.2539, -106.6721)
  spline S51 degree 2 poles (-175.2539, -106.6721) (-175.2539, -106.8474) (-175.4292, -106.8474) knots 0 0 0 1 1 1
  line L62 (-174.3805, -103.3474) -> (-173.5071, -103.3474)
  spline S52 degree 2 poles (-173.5071, -103.3474) (-173.0688, -103.3474) (-172.4584, -103.961) (-172.4584, -104.3961) knots 0 0 0 1 2 2 2
  spline S53 degree 2 poles (-172.4584, -104.3961) (-172.4584, -104.8636) (-173.0396, -105.4481) (-173.5071, -105.4481) knots 0 0 0 1 2 2 2
  line L63 (-173.5071, -105.4481) -> (-174.2052, -105.4481)
  line L64 (-174.2052, -105.4481) -> (-174.2052, -106.6721)
  spline S54 degree 2 poles (-174.2052, -106.6721) (-174.2052, -106.8474) (-174.3805, -106.8474) knots 0 0 0 1 1 1
  spline S55 degree 2 poles (-174.3805, -106.8474) (-174.5558, -106.8474) (-174.5558, -106.6721) knots 0 0 0 1 1 1
  line L65 (-174.5558, -106.6721) -> (-174.5558, -103.5227)
  spline S56 degree 2 poles (-174.5558, -103.5227) (-174.5558, -103.3474) (-174.3805, -103.3474) knots 0 0 0 1 1 1
  line L66 (-174.2052, -103.6981) -> (-174.2052, -105.0974)
  line L67 (-174.2052, -105.0974) -> (-173.5071, -105.0974)
  spline S57 degree 2 poles (-173.5071, -105.0974) (-173.2149, -105.0974) (-172.8091, -104.6916) (-172.8091, -104.3961) knots 0 0 0 1 2 2 2
  spline S58 degree 2 poles (-172.8091, -104.3961) (-172.8091, -104.1039) (-173.2149, -103.6981) (-173.5071, -103.6981) knots 0 0 0 1 2 2 2
  line L68 (-173.5071, -103.6981) -> (-174.2052, -103.6981)
  spline S59 degree 2 poles (-169.3091, -106.6721) (-169.3091, -106.8474) (-169.4844, -106.8474) knots 0 0 0 1 1 1
  spline S60 degree 2 poles (-169.4844, -106.8474) (-169.611, -106.8474) (-169.65, -106.7273) knots 0 0 0 1 1 1
  line L69 (-169.65, -106.7273) -> (-169.9032, -105.974)
  line L70 (-169.9032, -105.974) -> (-171.163, -105.974)
  line L71 (-171.163, -105.974) -> (-171.4162, -106.7273)
  spline S61 degree 2 poles (-171.4162, -106.7273) (-171.4552, -106.8474) (-171.5818, -106.8474) knots 0 0 0 1 1 1
  spline S62 degree 2 poles (-171.5818, -106.8474) (-171.7571, -106.8474) (-171.7571, -106.6721) knots 0 0 0 1 1 1
  spline S63 degree 2 poles (-171.7571, -106.6721) (-171.7571, -106.6396) (-171.7506, -106.6169) knots 0 0 0 1 1 1
  line L72 (-171.7506, -106.6169) -> (-170.7084, -103.487)
  spline S64 degree 2 poles (-170.7084, -103.487) (-170.6597, -103.3474) (-170.5331, -103.3474) knots 0 0 0 1 1 1
  spline S65 degree 2 poles (-170.5331, -103.3474) (-170.4065, -103.3474) (-170.361, -103.4838) knots 0 0 0 1 1 1
  line L73 (-170.361, -103.4838) -> (-169.3156, -106.6169)
  spline S66 degree 2 poles (-169.3156, -106.6169) (-169.3091, -106.6396) (-169.3091, -106.6721) knots 0 0 0 1 1 1
  line L74 (-170.5331, -104.0812) -> (-171.0461, -105.6234)
  line L75 (-171.0461, -105.6234) -> (-170.0201, -105.6234)
  line L76 (-170.0201, -105.6234) -> (-170.5331, -104.0812)
  spline S67 degree 2 poles (-168.6078, -103.5227) (-168.6078, -103.3474) (-168.4325, -103.3474) knots 0 0 0 1 1 1
  line L77 (-168.4325, -103.3474) -> (-167.3838, -103.3474)
  spline S68 degree 2 poles (-167.3838, -103.3474) (-167.0169, -103.3474) (-166.5104, -103.8539) (-166.5104, -104.2208) knots 0 0 0 1 2 2 2
  line L78 (-166.5104, -104.2208) -> (-166.5104, -105.9708)
  spline S69 degree 2 poles (-166.5104, -105.9708) (-166.5104, -106.3344) (-167.0201, -106.8474) (-167.3838, -106.8474) knots 0 0 0 1 2 2 2
  line L79 (-167.3838, -106.8474) -> (-168.4325, -106.8474)
  spline S70 degree 2 poles (-168.4325, -106.8474) (-168.6078, -106.8474) (-168.6078, -106.6721) knots 0 0 0 1 1 1
  line L80 (-168.6078, -106.6721) -> (-168.6078, -103.5227)
  line L81 (-168.2571, -103.6981) -> (-168.2571, -106.4968)
  line L82 (-168.2571, -106.4968) -> (-167.3838, -106.4968)
  spline S71 degree 2 poles (-167.3838, -106.4968) (-167.1662, -106.4968) (-166.861, -106.1883) (-166.861, -105.9708) knots 0 0 0 1 2 2 2
  line L83 (-166.861, -105.9708) -> (-166.861, -104.224)
  spline S72 degree 2 poles (-166.861, -104.224) (-166.861, -104.0065) (-167.1662, -103.6981) (-167.3838, -103.6981) knots 0 0 0 1 2 2 2
  line L84 (-167.3838, -103.6981) -> (-168.2571, -103.6981)
  spline S73 degree 2 poles (-163.7117, -105.7987) (-163.7117, -106.2338) (-164.3253, -106.8474) (-164.7604, -106.8474) knots 0 0 0 1 2 2 2
  spline S74 degree 2 poles (-164.7604, -106.8474) (-165.1955, -106.8474) (-165.8091, -106.2338) (-165.8091, -105.7987) knots 0 0 0 1 2 2 2
  line L85 (-165.8091, -105.7987) -> (-165.8091, -104.3961)
  spline S75 degree 2 poles (-165.8091, -104.3961) (-165.8091, -103.961) (-165.1955, -103.3474) (-164.7604, -103.3474) knots 0 0 0 1 2 2 2
  spline S76 degree 2 poles (-164.7604, -103.3474) (-164.3221, -103.3474) (-163.7117, -103.961) (-163.7117, -104.3961) knots 0 0 0 1 2 2 2
  line L86 (-163.7117, -104.3961) -> (-163.7117, -105.7987)
  line L87 (-164.0623, -105.7955) -> (-164.0623, -104.3961)
  spline S77 degree 2 poles (-164.0623, -104.3961) (-164.0623, -104.1039) (-164.4682, -103.6981) (-164.7604, -103.6981) knots 0 0 0 1 2 2 2
  spline S78 degree 2 poles (-164.7604, -103.6981) (-165.0526, -103.6981) (-165.4584, -104.1039) (-165.4584, -104.3961) knots 0 0 0 1 2 2 2
  line L88 (-165.4584, -104.3961) -> (-165.4584, -105.7955)
  spline S79 degree 2 poles (-165.4584, -105.7955) (-165.4584, -106.0909) (-165.0526, -106.4968) (-164.7604, -106.4968) knots 0 0 0 1 2 2 2
  spline S80 degree 2 poles (-164.7604, -106.4968) (-164.4682, -106.4968) (-164.0623, -106.0909) (-164.0623, -105.7955) knots 0 0 0 1 2 2 2
  line L89 (-161.5461, -105.3734) -> (-160.9357, -106.5942)
  spline S81 degree 2 poles (-160.9357, -106.5942) (-160.913, -106.6364) (-160.913, -106.6721) knots 0 0 0 1 1 1
  spline S82 degree 2 poles (-160.913, -106.6721) (-160.913, -106.7403) (-161.0201, -106.8474) (-161.0883, -106.8474) knots 0 0 0 1 2 2 2
  spline S83 degree 2 poles (-161.0883, -106.8474) (-161.1987, -106.8474) (-161.2474, -106.75) knots 0 0 0 1 1 1
  line L90 (-161.2474, -106.75) -> (-161.8968, -105.4448)
  spline S84 degree 2 poles (-161.8968, -105.4448) (-161.9227, -105.4481) (-161.9617, -105.4481) knots 0 0 0 1 1 1
  line L91 (-161.9617, -105.4481) -> (-162.6597, -105.4481)
  line L92 (-162.6597, -105.4481) -> (-162.6597, -106.6721)
  spline S85 degree 2 poles (-162.6597, -106.6721) (-162.6597, -106.8474) (-162.8351, -106.8474) knots 0 0 0 1 1 1
  spline S86 degree 2 poles (-162.8351, -106.8474) (-163.0104, -106.8474) (-163.0104, -106.6721) knots 0 0 0 1 1 1
  line L93 (-163.0104, -106.6721) -> (-163.0104, -103.5227)
  spline S87 degree 2 poles (-163.0104, -103.5227) (-163.0104, -103.3474) (-162.8351, -103.3474) knots 0 0 0 1 1 1
  line L94 (-162.8351, -103.3474) -> (-161.9617, -103.3474)
  spline S88 degree 2 poles (-161.9617, -103.3474) (-161.5234, -103.3474) (-160.913, -103.961) (-160.913, -104.3961) knots 0 0 0 1 2 2 2
  spline S89 degree 2 poles (-160.913, -104.3961) (-160.913, -105.1201) (-161.5461, -105.3734) knots 0 0 0 1 1 1
  line L95 (-162.6597, -103.6981) -> (-162.6597, -105.0974)
  line L96 (-162.6597, -105.0974) -> (-161.9617, -105.0974)
  spline S90 degree 2 poles (-161.9617, -105.0974) (-161.6695, -105.0974) (-161.2636, -104.6916) (-161.2636, -104.3961) knots 0 0 0 1 2 2 2
  spline S91 degree 2 poles (-161.2636, -104.3961) (-161.2636, -104.1039) (-161.6695, -103.6981) (-161.9617, -103.6981) knots 0 0 0 1 2 2 2
  line L97 (-161.9617, -103.6981) -> (-162.6597, -103.6981)
  line L98 (-157.2377, -106.4968) -> (-156.3643, -106.4968)
  line L99 (-156.3643, -106.4968) -> (-156.3643, -105.0974)
  line L100 (-156.3643, -105.0974) -> (-156.7149, -105.0974)
  spline S92 degree 2 poles (-156.7149, -105.0974) (-156.8903, -105.0974) (-156.8903, -104.9221) knots 0 0 0 1 1 1
  spline S93 degree 2 poles (-156.8903, -104.9221) (-156.8903, -104.7468) (-156.7149, -104.7468) knots 0 0 0 1 1 1
  line L101 (-156.7149, -104.7468) -> (-156.189, -104.7468)
  spline S94 degree 2 poles (-156.189, -104.7468) (-156.0136, -104.7468) (-156.0136, -104.9221) knots 0 0 0 1 1 1
  line L102 (-156.0136, -104.9221) -> (-156.0136, -106.6721)
  spline S95 degree 2 poles (-156.0136, -106.6721) (-156.0136, -106.8474) (-156.189, -106.8474) knots 0 0 0 1 1 1
  line L103 (-156.189, -106.8474) -> (-157.2377, -106.8474)
  spline S96 degree 2 poles (-157.2377, -106.8474) (-157.6013, -106.8474) (-158.111, -106.3344) (-158.111, -105.9708) knots 0 0 0 1 2 2 2
  line L104 (-158.111, -105.9708) -> (-158.111, -104.2208)
  spline S97 degree 2 poles (-158.111, -104.2208) (-158.111, -103.8604) (-157.6013, -103.3474) (-157.2377, -103.3474) knots 0 0 0 1 2 2 2
  line L105 (-157.2377, -103.3474) -> (-156.189, -103.3474)
  spline S98 degree 2 poles (-156.189, -103.3474) (-156.0136, -103.3474) (-156.0136, -103.5227) knots 0 0 0 1 1 1
  spline S99 degree 2 poles (-156.0136, -103.5227) (-156.0136, -103.6981) (-156.189, -103.6981) knots 0 0 0 1 1 1
  line L106 (-156.189, -103.6981) -> (-157.2377, -103.6981)
  spline S100 degree 2 poles (-157.2377, -103.6981) (-157.4552, -103.6981) (-157.7604, -104.0065) (-157.7604, -104.224) knots 0 0 0 1 2 2 2
  line L107 (-157.7604, -104.224) -> (-157.7604, -105.9708)
  spline S101 degree 2 poles (-157.7604, -105.9708) (-157.7604, -106.1916) (-157.4552, -106.4968) (-157.2377, -106.4968) knots 0 0 0 1 2 2 2
  line L108 (-152.3383, -106.4968) -> (-151.4649, -106.4968)
  line L109 (-151.4649, -106.4968) -> (-151.4649, -105.0974)
  line L110 (-151.4649, -105.0974) -> (-151.8156, -105.0974)
  spline S102 degree 2 poles (-151.8156, -105.0974) (-151.9909, -105.0974) (-151.9909, -104.9221) knots 0 0 0 1 1 1
  spline S103 degree 2 poles (-151.9909, -104.9221) (-151.9909, -104.7468) (-151.8156, -104.7468) knots 0 0 0 1 1 1
  line L111 (-151.8156, -104.7468) -> (-151.2896, -104.7468)
  spline S104 degree 2 poles (-151.2896, -104.7468) (-151.1143, -104.7468) (-151.1143, -104.9221) knots 0 0 0 1 1 1
  line L112 (-151.1143, -104.9221) -> (-151.1143, -106.6721)
  spline S105 degree 2 poles (-151.1143, -106.6721) (-151.1143, -106.8474) (-151.2896, -106.8474) knots 0 0 0 1 1 1
  line L113 (-151.2896, -106.8474) -> (-152.3383, -106.8474)
  spline S106 degree 2 poles (-152.3383, -106.8474) (-152.7019, -106.8474) (-153.2117, -106.3344) (-153.2117, -105.9708) knots 0 0 0 1 2 2 2
  line L114 (-153.2117, -105.9708) -> (-153.2117, -104.2208)
  spline S107 degree 2 poles (-153.2117, -104.2208) (-153.2117, -103.8604) (-152.7019, -103.3474) (-152.3383, -103.3474) knots 0 0 0 1 2 2 2
  line L115 (-152.3383, -103.3474) -> (-151.2896, -103.3474)
  spline S108 degree 2 poles (-151.2896, -103.3474) (-151.1143, -103.3474) (-151.1143, -103.5227) knots 0 0 0 1 1 1
  spline S109 degree 2 poles (-151.1143, -103.5227) (-151.1143, -103.6981) (-151.2896, -103.6981) knots 0 0 0 1 1 1
  line L116 (-151.2896, -103.6981) -> (-152.3383, -103.6981)
  spline S110 degree 2 poles (-152.3383, -103.6981) (-152.5558, -103.6981) (-152.861, -104.0065) (-152.861, -104.224) knots 0 0 0 1 2 2 2
  line L117 (-152.861, -104.224) -> (-152.861, -105.9708)
  spline S111 degree 2 poles (-152.861, -105.9708) (-152.861, -106.1916) (-152.5558, -106.4968) (-152.3383, -106.4968) knots 0 0 0 1 2 2 2
  line L118 (-148.9487, -105.3734) -> (-148.3383, -106.5942)
  spline S112 degree 2 poles (-148.3383, -106.5942) (-148.3156, -106.6364) (-148.3156, -106.6721) knots 0 0 0 1 1 1
  spline S113 degree 2 poles (-148.3156, -106.6721) (-148.3156, -106.7403) (-148.4227, -106.8474) (-148.4909, -106.8474) knots 0 0 0 1 2 2 2
  spline S114 degree 2 poles (-148.4909, -106.8474) (-148.6013, -106.8474) (-148.65, -106.75) knots 0 0 0 1 1 1
  line L119 (-148.65, -106.75) -> (-149.2994, -105.4448)
  spline S115 degree 2 poles (-149.2994, -105.4448) (-149.3253, -105.4481) (-149.3643, -105.4481) knots 0 0 0 1 1 1
  line L120 (-149.3643, -105.4481) -> (-150.0623, -105.4481)
  line L121 (-150.0623, -105.4481) -> (-150.0623, -106.6721)
  spline S116 degree 2 poles (-150.0623, -106.6721) (-150.0623, -106.8474) (-150.2377, -106.8474) knots 0 0 0 1 1 1
  spline S117 degree 2 poles (-150.2377, -106.8474) (-150.413, -106.8474) (-150.413, -106.6721) knots 0 0 0 1 1 1
  line L122 (-150.413, -106.6721) -> (-150.413, -103.5227)
  spline S118 degree 2 poles (-150.413, -103.5227) (-150.413, -103.3474) (-150.2377, -103.3474) knots 0 0 0 1 1 1
  line L123 (-150.2377, -103.3474) -> (-149.3643, -103.3474)
  spline S119 degree 2 poles (-149.3643, -103.3474) (-148.926, -103.3474) (-148.3156, -103.961) (-148.3156, -104.3961) knots 0 0 0 1 2 2 2
  spline S120 degree 2 poles (-148.3156, -104.3961) (-148.3156, -105.1201) (-148.9487, -105.3734) knots 0 0 0 1 1 1
  line L124 (-150.0623, -103.6981) -> (-150.0623, -105.0974)
  line L125 (-150.0623, -105.0974) -> (-149.3643, -105.0974)
  spline S121 degree 2 poles (-149.3643, -105.0974) (-149.0721, -105.0974) (-148.6662, -104.6916) (-148.6662, -104.3961) knots 0 0 0 1 2 2 2
  spline S122 degree 2 poles (-148.6662, -104.3961) (-148.6662, -104.1039) (-149.0721, -103.6981) (-149.3643, -103.6981) knots 0 0 0 1 2 2 2
  line L126 (-149.3643, -103.6981) -> (-150.0623, -103.6981)
  line L127 (-146.2149, -103.5227) -> (-146.2149, -105.9708)
  spline S123 degree 2 poles (-146.2149, -105.9708) (-146.2149, -106.3377) (-146.7279, -106.8474) (-147.0916, -106.8474) knots 0 0 0 1 2 2 2
  line L128 (-147.0916, -106.8474) -> (-147.439, -106.8474)
  spline S124 degree 2 poles (-147.439, -106.8474) (-147.6143, -106.8474) (-147.6143, -106.6721) knots 0 0 0 1 1 1
  spline S125 degree 2 poles (-147.6143, -106.6721) (-147.6143, -106.4968) (-147.439, -106.4968) knots 0 0 0 1 1 1
  line L129 (-147.439, -106.4968) -> (-147.0916, -106.4968)
  spline S126 degree 2 poles (-147.0916, -106.4968) (-146.8708, -106.4968) (-146.5656, -106.1883) (-146.5656, -105.9708) knots 0 0 0 1 2 2 2
  line L130 (-146.5656, -105.9708) -> (-146.5656, -103.5227)
  spline S127 degree 2 poles (-146.5656, -103.5227) (-146.5656, -103.3474) (-146.3903, -103.3474) knots 0 0 0 1 1 1
  spline S128 degree 2 poles (-146.3903, -103.3474) (-146.2149, -103.3474) (-146.2149, -103.5227) knots 0 0 0 1 1 1
  line L131 (-143.2734, -106.0162) -> (-142.7117, -103.4838)
  spline S129 degree 2 poles (-142.7117, -103.4838) (-142.6792, -103.3474) (-142.5396, -103.3474) knots 0 0 0 1 1 1
  spline S130 degree 2 poles (-142.5396, -103.3474) (-142.3643, -103.3474) (-142.3643, -103.5227) knots 0 0 0 1 1 1
  spline S131 degree 2 poles (-142.3643, -103.5227) (-142.3643, -103.539) (-142.3708, -103.5617) knots 0 0 0 1 1 1
  line L132 (-142.3708, -103.5617) -> (-143.0688, -106.7013)